vape_naysh (Autodesk Fusion 360 design; units mm, degrees)
Autodesk Fusion 360 part; units mm, degrees
(part 1 of 3)
sketch "Sketch1" plane through (0, 0, 0) normal (0, 1, 0) x (1, 0, 0)
  line L0 (3, -30) -> (14, -30)
  line L1 (14, -30) -> (16, -17)
  line L2 (16, -17) -> (19.2504, -13.3707)
  line L3 (19.2504, -13.3707) -> (19.2504, 30)
  line L4 (19.2504, 30) -> (15, 34.5)
  line L5 (15, 34.5) -> (-12.65, 34.5)
  line L6 (-12.65, 34.5) -> (-16.7887, 30.816)
  line L7 (-16.7887, 30.816) -> (-16.7887, -12.5)
  line L8 (-16.7887, -12.5) -> (-14, -16.5)
  line L9 (-14, -16.5) -> (-1, -16.5)
  line L10 (-1, -16.5) -> (1.175, -18.2567)
  line L11 (1.175, -18.2567) -> (3, -30)
  line L12 (14.6863, -30.8) -> (16.7545, -17.3566)
  line L13 (16.7545, -17.3566) -> (20.0504, -13.6766)
  line L14 (20.0504, -13.6766) -> (20.0504, 30.3181)
  line L15 (20.0504, 30.3181) -> (15.3448, 35.3)
  line L16 (15.3448, 35.3) -> (-12.9545, 35.3)
  line L17 (-12.9545, 35.3) -> (-17.5887, 31.1749)
  line L18 (-17.5887, 31.1749) -> (-17.5887, -12.7513)
  line L19 (-17.5887, -12.7513) -> (-14.4175, -17.3)
  line L20 (-14.4175, -17.3) -> (-1.2827, -17.3)
  line L21 (-1.2827, -17.3) -> (0.4319, -18.6849)
  line L22 (0.4319, -18.6849) -> (2.3147, -30.8)
  line L23 (2.3147, -30.8) -> (14.6863, -30.8)
  dimension "d1" = 0.8
  constraint horizontal L0
  constraint perpendicular L0 L3
  constraint perpendicular L3 L5
  constraint perpendicular L5 L7
  constraint perpendicular L3 L9
sketch "Sketch2" plane through (0, 0, 0) normal (0, 1, 0) x (1, 0, 0)
  spline S0 degree 3 poles (-4.3083, 22.4434) (-8.6322, 22.1667) (-11.0016, 21.717) (-11.5724, 21.0771) knots 0 0 0 0 1 1 1 1
  spline S1 degree 3 poles (-11.5724, 21.0771) (-11.7799, 20.8349) (-11.8491, 20.5236) (-11.8145, 19.9183) knots 0 0 0 0 1 1 1 1
  spline S2 degree 3 poles (-11.8145, 19.9183) (-11.7626, 19.1054) (-11.728, 19.0535) (-10.9843, 18.6903) knots 0 0 0 0 1 1 1 1
  spline S3 degree 3 poles (-10.9843, 18.6903) (-10.2579, 18.3271) (-9.3067, 18.1714) (-4.6715, 17.6526) knots 0 0 0 0 1 1 1 1
  line L0 (-4.6715, 17.6526) -> (-3.4608, 17.5142)
  line L1 (-3.4608, 17.5142) -> (-2.9074, 16.1306)
  spline S4 degree 3 poles (-2.9074, 16.1306) (-2.6133, 15.3696) (-2.3193, 14.4875) (-2.2501, 14.1935) knots 0 0 0 0 1 1 1 1
  line L2 (-2.2501, 14.1935) -> (-2.1291, 13.6228)
  line L3 (-2.1291, 13.6228) -> (-3.236, 13.6228)
  spline S5 degree 3 poles (-3.236, 13.6228) (-4.5331, 13.6228) (-7.7674, 13.2077) (-8.4073, 12.9655) knots 0 0 0 0 1 1 1 1
  spline S6 degree 3 poles (-8.4073, 12.9655) (-9.1337, 12.6715) (-9.4277, 12.2737) (-9.4277, 11.53) knots 0 0 0 0 1 1 1 1
  spline S7 degree 3 poles (-9.4277, 11.53) (-9.4277, 10.1291) (-8.3381, 9.7659) (-2.9766, 9.3681) knots 0 0 0 0 1 1 1 1
  spline S8 degree 3 poles (-2.9766, 9.3681) (-2.1464, 9.3162) (-1.4719, 9.1951) (-1.4719, 9.1259) knots 0 0 0 0 1 1 1 1
  spline S9 degree 3 poles (-1.4719, 9.1259) (-1.4719, 9.0395) (-1.8351, 9.0049) (-2.2847, 9.0741) knots 0 0 0 0 1 1 1 1
  spline S10 degree 3 poles (-2.2847, 9.0741) (-3.4435, 9.1951) (-4.5504, 8.8665) (-5.2077, 8.1747) knots 0 0 0 0 1 1 1 1
  spline S11 degree 3 poles (-5.2077, 8.1747) (-5.7092, 7.6385) (-5.813, 7.6039) (-7.1102, 7.5521) knots 0 0 0 0 1 1 1 1
  spline S12 degree 3 poles (-7.1102, 7.5521) (-8.2862, 7.5002) (-8.6149, 7.4137) (-9.2375, 6.9986) knots 0 0 0 0 1 1 1 1
  spline S13 degree 3 poles (-9.2375, 6.9986) (-10.0158, 6.4797) (-10.6211, 5.4247) (-10.6384, 4.6118) knots 0 0 0 0 1 1 1 1
  spline S14 degree 3 poles (-10.6384, 4.6118) (-10.6384, 4.3524) (-10.7595, 4.0584) (-10.9152, 3.92) knots 0 0 0 0 1 1 1 1
  spline S15 degree 3 poles (-10.9152, 3.92) (-11.5724, 3.3666) (-11.9183, 2.3288) (-11.9356, 0.8241) knots 0 0 0 0 1 1 1 1
  spline S16 degree 3 poles (-11.9356, 0.8241) (-11.9356, -0.94) (-11.607, -1.7529) (-10.6211, -2.4447) knots 0 0 0 0 1 1 1 1
  spline S17 degree 3 poles (-10.6211, -2.4447) (-10.2579, -2.6868) (-9.9639, -3.0154) (-9.9466, -3.1538) knots 0 0 0 0 1 1 1 1
  spline S18 degree 3 poles (-9.9466, -3.1538) (-9.9466, -3.2922) (-9.7909, -3.6727) (-9.6007, -3.984) knots 0 0 0 0 1 1 1 1
  spline S19 degree 3 poles (-9.6007, -3.984) (-9.4104, -4.2953) (-9.2548, -4.7277) (-9.2548, -4.9352) knots 0 0 0 0 1 1 1 1
  spline S20 degree 3 poles (-9.2548, -4.9352) (-9.2548, -5.506) (-8.4938, -6.5264) (-7.8193, -6.855) knots 0 0 0 0 1 1 1 1
  spline S21 degree 3 poles (-7.8193, -6.855) (-7.4907, -7.0107) (-6.8334, -7.1317) (-6.3665, -7.1317) knots 0 0 0 0 1 1 1 1
  spline S22 degree 3 poles (-6.3665, -7.1317) (-5.9168, -7.1317) (-5.225, -7.2528) (-4.8445, -7.3912) knots 0 0 0 0 1 1 1 1
  spline S23 degree 3 poles (-4.8445, -7.3912) (-4.464, -7.5295) (-3.9105, -7.6333) (-3.6165, -7.6506) knots 0 0 0 0 1 1 1 1
  spline S24 degree 3 poles (-3.6165, -7.6506) (-3.3052, -7.6506) (-3.0284, -7.7544) (-2.9766, -7.8927) knots 0 0 0 0 1 1 1 1
  spline S25 degree 3 poles (-2.9766, -7.8927) (-2.9247, -8.0311) (-2.5096, -8.3597) (-2.0426, -8.6364) knots 0 0 0 0 1 1 1 1
  spline S26 degree 3 poles (-2.0426, -8.6364) (-1.2989, -9.0688) (-1.0395, -9.1207) (0.2577, -9.1207) knots 0 0 0 0 1 1 1 1
  spline S27 degree 3 poles (0.2577, -9.1207) (1.9008, -9.1207) (2.4888, -8.8959) (3.4919, -7.8927) knots 0 0 0 0 1 1 1 1
  spline S28 degree 3 poles (3.4919, -7.8927) (3.8033, -7.5641) (4.2356, -7.3047) (4.4259, -7.3047) knots 0 0 0 0 1 1 1 1
  spline S29 degree 3 poles (4.4259, -7.3047) (4.6334, -7.3047) (5.2388, -7.0799) (5.7749, -6.8031) knots 0 0 0 0 1 1 1 1
  spline S30 degree 3 poles (5.7749, -6.8031) (6.5013, -6.4226) (7.0721, -6.267) (8.0406, -6.1978) knots 0 0 0 0 1 1 1 1
  spline S31 degree 3 poles (8.0406, -6.1978) (10.4966, -6.0075) (11.7591, -5.8173) (12.1223, -5.5925) knots 0 0 0 0 1 1 1 1
  spline S32 degree 3 poles (12.1223, -5.5925) (12.745, -5.1947) (13.0909, -4.3991) (13.2465, -3.05) knots 0 0 0 0 1 1 1 1
  spline S33 degree 3 poles (13.2465, -3.05) (13.3676, -2.0988) (13.5579, -1.5626) (13.973, -0.8881) knots 0 0 0 0 1 1 1 1
  spline S34 degree 3 poles (13.973, -0.8881) (14.4918, -0.0579) (14.5264, 0.1323) (14.5264, 1.516) knots 0 0 0 0 1 1 1 1
  spline S35 degree 3 poles (14.5264, 1.516) (14.5264, 2.865) (14.4745, 3.0898) (14.0594, 3.7298) knots 0 0 0 0 1 1 1 1
  spline S36 degree 3 poles (14.0594, 3.7298) (13.8, 4.1276) (13.2638, 4.6291) (12.8833, 4.8367) knots 0 0 0 0 1 1 1 1
  spline S37 degree 3 poles (12.8833, 4.8367) (12.451, 5.0961) (12.1915, 5.3555) (12.1915, 5.5804) knots 0 0 0 0 1 1 1 1
  spline S38 degree 3 poles (12.1915, 5.5804) (12.1915, 6.1165) (11.5689, 7.0159) (10.9463, 7.4137) knots 0 0 0 0 1 1 1 1
  spline S39 degree 3 poles (10.9463, 7.4137) (10.4447, 7.7077) (10.1853, 7.7423) (8.8189, 7.6731) knots 0 0 0 0 1 1 1 1
  spline S40 degree 3 poles (8.8189, 7.6731) (6.5359, 7.5348) (5.5501, 7.5694) (5.4117, 7.7942) knots 0 0 0 0 1 1 1 1
  spline S41 degree 3 poles (5.4117, 7.7942) (5.3425, 7.9153) (5.2734, 8.2785) (5.2734, 8.6417) knots 0 0 0 0 1 1 1 1
  line L4 (5.2734, 8.6417) -> (5.2734, 9.2643)
  line L5 (5.2734, 9.2643) -> (6.6224, 9.3681)
  spline S42 degree 3 poles (6.6224, 9.3681) (11.3613, 9.7486) (12.5374, 10.1637) (12.5374, 11.4781) knots 0 0 0 0 1 1 1 1
  spline S43 degree 3 poles (12.5374, 11.4781) (12.5374, 12.3083) (12.2953, 12.6888) (11.6381, 12.9136) knots 0 0 0 0 1 1 1 1
  spline S44 degree 3 poles (11.6381, 12.9136) (10.8771, 13.1904) (7.8331, 13.6228) (6.6916, 13.6228) knots 0 0 0 0 1 1 1 1
  spline S45 degree 3 poles (6.6916, 13.6228) (5.896, 13.6228) (5.7749, 13.6573) (5.8441, 13.9341) knots 0 0 0 0 1 1 1 1
  spline S46 degree 3 poles (5.8441, 13.9341) (6.2938, 15.5425) (6.7089, 16.7359) (7.0029, 17.2202) knots 0 0 0 0 1 1 1 1
  spline S47 degree 3 poles (7.0029, 17.2202) (7.3142, 17.7218) (7.418, 17.7737) (8.1617, 17.7737) knots 0 0 0 0 1 1 1 1
  spline S48 degree 3 poles (8.1617, 17.7737) (9.1994, 17.7737) (12.3472, 18.2233) (13.2465, 18.4828) knots 0 0 0 0 1 1 1 1
  spline S49 degree 3 poles (13.2465, 18.4828) (14.2324, 18.7941) (14.4745, 19.1227) (14.4053, 20.2123) knots 0 0 0 0 1 1 1 1
  spline S50 degree 3 poles (14.4053, 20.2123) (14.3535, 21.0252) (14.3016, 21.1636) (13.8865, 21.3711) knots 0 0 0 0 1 1 1 1
  spline S51 degree 3 poles (13.8865, 21.3711) (13.2465, 21.6651) (11.4478, 22.0283) (9.4243, 22.2705) knots 0 0 0 0 1 1 1 1
  spline S52 degree 3 poles (9.4243, 22.2705) (7.245, 22.5126) (-1.5064, 22.6337) (-4.3083, 22.4434) knots 0 0 0 0 1 1 1 1
  spline S53 degree 3 poles (5.2734, 20.368) (6.2765, 20.3161) (6.8818, 20.2469) (6.6397, 20.2296) knots 0 0 0 0 1 1 1 1
  spline S54 degree 3 poles (6.6397, 20.2296) (5.8787, 20.1777) (5.1004, 19.1227) (4.3913, 17.1856) knots 0 0 0 0 1 1 1 1
  line L6 (4.3913, 17.1856) -> (4.0627, 16.3035)
  line L7 (4.0627, 16.3035) -> (4.1665, 17.1164)
  spline S55 degree 3 poles (4.1665, 17.1164) (4.2356, 17.5661) (4.2183, 18.1369) (4.1665, 18.379) knots 0 0 0 0 1 1 1 1
  spline S56 degree 3 poles (4.1665, 18.379) (4.0627, 18.7768) (3.9762, 18.8114) (3.1979, 18.8114) knots 0 0 0 0 1 1 1 1
  spline S57 degree 3 poles (3.1979, 18.8114) (2.4196, 18.8114) (2.2985, 18.7595) (2.1602, 18.3617) knots 0 0 0 0 1 1 1 1
  spline S58 degree 3 poles (2.1602, 18.3617) (2.0564, 18.1196) (1.9872, 17.7045) (1.9872, 17.4277) knots 0 0 0 0 1 1 1 1
  spline S59 degree 3 poles (1.9872, 17.4277) (1.9872, 17.151) (1.918, 16.8916) (1.8316, 16.8397) knots 0 0 0 0 1 1 1 1
  spline S60 degree 3 poles (1.8316, 16.8397) (1.7624, 16.7878) (1.6413, 17.4104) (1.5721, 18.2406) knots 0 0 0 0 1 1 1 1
  spline S61 degree 3 poles (1.5721, 18.2406) (1.3992, 20.2469) (1.3127, 20.4026) (0.2923, 20.3334) knots 0 0 0 0 1 1 1 1
  line L8 (0.2923, 20.3334) -> (-0.5206, 20.2815)
  line L9 (-0.5206, 20.2815) -> (-0.486, 18.4136)
  line L10 (-0.486, 18.4136) -> (-0.4687, 16.5284)
  line L11 (-0.4687, 16.5284) -> (-1.0395, 17.8428)
  spline S62 degree 3 poles (-1.0395, 17.8428) (-1.3508, 18.5519) (-1.7659, 19.4167) (-1.9561, 19.7453) knots 0 0 0 0 1 1 1 1
  line L12 (-1.9561, 19.7453) -> (-2.3193, 20.3507)
  line L13 (-2.3193, 20.3507) -> (-1.7659, 20.4198)
  spline S63 degree 3 poles (-1.7659, 20.4198) (-0.8492, 20.5236) (3.3363, 20.5063) (5.2734, 20.368) knots 0 0 0 0 1 1 1 1
  spline S64 degree 3 poles (-4.1008, 20.1604) (-4.2045, 19.8491) (-4.6542, 19.7972) (-5.6055, 19.9529) knots 0 0 0 0 1 1 1 1
  line L14 (-5.6055, 19.9529) -> (-6.401, 20.0912)
  line L15 (-6.401, 20.0912) -> (-5.3633, 20.2123)
  spline S65 degree 3 poles (-5.3633, 20.2123) (-4.7926, 20.2642) (-4.2564, 20.3161) (-4.1872, 20.3334) knots 0 0 0 0 1 1 1 1
  spline S66 degree 3 poles (-4.1872, 20.3334) (-4.1008, 20.3507) (-4.0662, 20.2642) (-4.1008, 20.1604) knots 0 0 0 0 1 1 1 1
  spline S67 degree 3 poles (8.8189, 20.0221) (8.767, 19.9356) (8.4903, 19.8491) (8.2136, 19.8491) knots 0 0 0 0 1 1 1 1
  spline S68 degree 3 poles (8.2136, 19.8491) (7.9369, 19.8491) (7.6601, 19.9356) (7.6082, 20.0221) knots 0 0 0 0 1 1 1 1
  spline S69 degree 3 poles (7.6082, 20.0221) (7.5391, 20.1258) (7.7812, 20.195) (8.2136, 20.195) knots 0 0 0 0 1 1 1 1
  spline S70 degree 3 poles (8.2136, 20.195) (8.646, 20.195) (8.8881, 20.1258) (8.8189, 20.0221) knots 0 0 0 0 1 1 1 1
  spline S71 degree 3 poles (1.4684, 9.2297) (1.4684, 8.6936) (1.3819, 8.4341) (1.1916, 8.3649) knots 0 0 0 0 1 1 1 1
  spline S72 degree 3 poles (1.1916, 8.3649) (0.6728, 8.1747) (0.6036, 8.2612) (0.6036, 9.1259) knots 0 0 0 0 1 1 1 1
  spline S73 degree 3 poles (0.6036, 9.1259) (0.6036, 9.9388) (0.6382, 9.9907) (1.036, 9.9907) knots 0 0 0 0 1 1 1 1
  spline S74 degree 3 poles (1.036, 9.9907) (1.4338, 9.9907) (1.4684, 9.9215) (1.4684, 9.2297) knots 0 0 0 0 1 1 1 1
  spline S75 degree 3 poles (-0.2266, 5.148) (-0.2612, 4.7502) (-0.2093, 4.3351) (-0.0882, 4.1967) knots 0 0 0 0 1 1 1 1
  spline S76 degree 3 poles (-0.0882, 4.1967) (0.2404, 3.8163) (1.3473, 3.8681) (1.8835, 4.3005) knots 0 0 0 0 1 1 1 1
  spline S77 degree 3 poles (1.8835, 4.3005) (2.3504, 4.6637) (2.3677, 4.6637) (2.8001, 4.3524) knots 0 0 0 0 1 1 1 1
  spline S78 degree 3 poles (2.8001, 4.3524) (3.0423, 4.1622) (3.3363, 3.7471) (3.44, 3.4185) knots 0 0 0 0 1 1 1 1
  spline S79 degree 3 poles (3.44, 3.4185) (3.6303, 2.8304) (3.6649, 2.8131) (4.4951, 2.8131) knots 0 0 0 0 1 1 1 1
  line L16 (4.4951, 2.8131) -> (5.3598, 2.8131)
  line L17 (5.3598, 2.8131) -> (5.4117, 3.799)
  spline S80 degree 3 poles (5.4117, 3.799) (5.4463, 4.3524) (5.3771, 4.9577) (5.2734, 5.148) knots 0 0 0 0 1 1 1 1
  spline S81 degree 3 poles (5.2734, 5.148) (5.135, 5.4247) (5.135, 5.4939) (5.3425, 5.4939) knots 0 0 0 0 1 1 1 1
  spline S82 degree 3 poles (5.3425, 5.4939) (6.2073, 5.4939) (7.8504, 4.2486) (7.5045, 3.8335) knots 0 0 0 0 1 1 1 1
  spline S83 degree 3 poles (7.5045, 3.8335) (7.418, 3.7125) (7.3488, 3.2455) (7.3834, 2.7785) knots 0 0 0 0 1 1 1 1
  line L18 (7.3834, 2.7785) -> (7.4353, 1.9483)
  line L19 (7.4353, 1.9483) -> (8.2309, 1.8965)
  spline S84 degree 3 poles (8.2309, 1.8965) (8.94, 1.8446) (9.0956, 1.9138) (9.6491, 2.4672) knots 0 0 0 0 1 1 1 1
  spline S85 degree 3 poles (9.6491, 2.4672) (10.4793, 3.2974) (11.1019, 3.2974) (11.8629, 2.4326) knots 0 0 0 0 1 1 1 1
  line L20 (11.8629, 2.4326) -> (12.4337, 1.7754)
  line L21 (12.4337, 1.7754) -> (11.4478, 1.7235)
  line L22 (11.4478, 1.7235) -> (10.462, 1.6716)
  line L23 (10.462, 1.6716) -> (10.462, 0.8241)
  spline S86 degree 3 poles (10.462, 0.8241) (10.462, 0.1496) (10.5485, -0.1098) (10.8944, -0.4557) knots 0 0 0 0 1 1 1 1
  spline S87 degree 3 poles (10.8944, -0.4557) (11.4305, -0.9919) (11.4305, -1.2686) (10.9463, -1.7356) knots 0 0 0 0 1 1 1 1
  spline S88 degree 3 poles (10.9463, -1.7356) (10.6522, -1.995) (10.2717, -2.1161) (9.5972, -2.1507) knots 0 0 0 0 1 1 1 1
  line L24 (9.5972, -2.1507) -> (8.646, -2.2026)
  line L25 (8.646, -2.2026) -> (8.5595, -3.1538)
  spline S89 degree 3 poles (8.5595, -3.1538) (8.473, -4.0359) (8.4384, -4.1051) (7.9023, -4.2607) knots 0 0 0 0 1 1 1 1
  spline S90 degree 3 poles (7.9023, -4.2607) (7.1759, -4.4683) (7.0894, -4.3472) (7.4353, -3.6727) knots 0 0 0 0 1 1 1 1
  spline S91 degree 3 poles (7.4353, -3.6727) (7.6082, -3.3268) (7.6947, -2.8252) (7.6601, -2.2371) knots 0 0 0 0 1 1 1 1
  line L26 (7.6601, -2.2371) -> (7.6082, -1.3378)
  line L27 (7.6082, -1.3378) -> (6.7262, -1.2859)
  spline S92 degree 3 poles (6.7262, -1.2859) (5.896, -1.234) (5.8441, -1.2513) (5.602, -1.7875) knots 0 0 0 0 1 1 1 1
  spline S93 degree 3 poles (5.602, -1.7875) (5.4809, -2.0988) (5.1523, -2.4966) (4.8929, -2.6868) knots 0 0 0 0 1 1 1 1
  spline S94 degree 3 poles (4.8929, -2.6868) (4.4605, -3.0154) (4.4086, -3.0154) (3.9935, -2.756) knots 0 0 0 0 1 1 1 1
  spline S95 degree 3 poles (3.9935, -2.756) (3.7514, -2.5831) (3.2152, -2.462) (2.7828, -2.462) knots 0 0 0 0 1 1 1 1
  spline S96 degree 3 poles (2.7828, -2.462) (1.9526, -2.462) (1.8143, -2.6176) (1.8143, -3.5689) knots 0 0 0 0 1 1 1 1
  spline S97 degree 3 poles (1.8143, -3.5689) (1.8143, -4.2607) (2.2121, -4.6585) (3.2325, -4.9698) knots 0 0 0 0 1 1 1 1
  line L28 (3.2325, -4.9698) -> (3.9762, -5.1774)
  line L29 (3.9762, -5.1774) -> (3.3363, -5.3676)
  spline S98 degree 3 poles (3.3363, -5.3676) (2.9904, -5.4541) (2.4542, -5.4887) (2.1429, -5.4195) knots 0 0 0 0 1 1 1 1
  line L30 (2.1429, -5.4195) -> (1.5721, -5.2984)
  line L31 (1.5721, -5.2984) -> (1.624, -4.2434)
  spline S99 degree 3 poles (1.624, -4.2434) (1.6586, -3.223) (1.6413, -3.1538) (1.2435, -3.0673) knots 0 0 0 0 1 1 1 1
  spline S100 degree 3 poles (1.2435, -3.0673) (0.4134, -2.8598) (-0.1574, -3.0327) (-0.4168, -3.5862) knots 0 0 0 0 1 1 1 1
  spline S101 degree 3 poles (-0.4168, -3.5862) (-1.0741, -5.0217) (-2.475, -5.8173) (-3.5473, -5.3503) knots 0 0 0 0 1 1 1 1
  line L32 (-3.5473, -5.3503) -> (-4.1526, -5.0909)
  line L33 (-4.1526, -5.0909) -> (-3.5127, -5.0736)
  spline S102 degree 3 poles (-3.5127, -5.0736) (-3.1668, -5.0563) (-2.6652, -4.9698) (-2.4231, -4.8488) knots 0 0 0 0 1 1 1 1
  spline S103 degree 3 poles (-2.4231, -4.8488) (-2.008, -4.6585) (-1.9734, -4.572) (-2.0253, -3.7764) knots 0 0 0 0 1 1 1 1
  line L34 (-2.0253, -3.7764) -> (-2.0772, -2.8944)
  line L35 (-2.0772, -2.8944) -> (-3.1668, -2.8771)
  spline S104 degree 3 poles (-3.1668, -2.8771) (-4.4294, -2.8425) (-4.8963, -2.5312) (-5.0866, -1.5799) knots 0 0 0 0 1 1 1 1
  spline S105 degree 3 poles (-5.0866, -1.5799) (-5.1904, -1.0265) (-5.2422, -0.9919) (-6.0378, -0.94) knots 0 0 0 0 1 1 1 1
  spline S106 degree 3 poles (-6.0378, -0.94) (-6.4875, -0.9054) (-6.9718, -0.9746) (-7.0929, -1.0784) knots 0 0 0 0 1 1 1 1
  spline S107 degree 3 poles (-7.0929, -1.0784) (-7.4734, -1.3897) (-8.3554, -1.1129) (-8.9954, -0.4557) knots 0 0 0 0 1 1 1 1
  spline S108 degree 3 poles (-8.9954, -0.4557) (-9.7909, 0.3226) (-9.912, 0.8933) (-9.4969, 1.6716) knots 0 0 0 0 1 1 1 1
  spline S109 degree 3 poles (-9.4969, 1.6716) (-8.9608, 2.6402) (-8.4246, 2.9342) (-7.0756, 2.9688) knots 0 0 0 0 1 1 1 1
  line L36 (-7.0756, 2.9688) -> (-5.8822, 2.9861)
  line L37 (-5.8822, 2.9861) -> (-5.8303, 3.7817)
  spline S110 degree 3 poles (-5.8303, 3.7817) (-5.7784, 4.4908) (-5.7092, 4.6291) (-5.2768, 4.8021) knots 0 0 0 0 1 1 1 1
  spline S111 degree 3 poles (-5.2768, 4.8021) (-4.8963, 4.9577) (-4.7061, 4.9577) (-4.3429, 4.7675) knots 0 0 0 0 1 1 1 1
  line L38 (-4.3429, 4.7675) -> (-3.8932, 4.5254)
  line L39 (-3.8932, 4.5254) -> (-4.4985, 4.214)
  spline S112 degree 3 poles (-4.4985, 4.214) (-5.1904, 3.8335) (-5.7957, 2.7439) (-5.7957, 1.8446) knots 0 0 0 0 1 1 1 1
  spline S113 degree 3 poles (-5.7957, 1.8446) (-5.7957, 1.0836) (-5.5363, 0.8241) (-4.758, 0.8241) knots 0 0 0 0 1 1 1 1
  spline S114 degree 3 poles (-4.758, 0.8241) (-4.0316, 0.8241) (-3.8932, 0.9279) (-3.5473, 1.5851) knots 0 0 0 0 1 1 1 1
  spline S115 degree 3 poles (-3.5473, 1.5851) (-3.4089, 1.8619) (-3.1149, 2.1905) (-2.9247, 2.3288) knots 0 0 0 0 1 1 1 1
  spline S116 degree 3 poles (-2.9247, 2.3288) (-2.596, 2.5364) (-2.4923, 2.5191) (-2.0253, 2.1213) knots 0 0 0 0 1 1 1 1
  spline S117 degree 3 poles (-2.0253, 2.1213) (-1.4546, 1.6543) (-0.3304, 1.516) (0.0501, 1.8965) knots 0 0 0 0 1 1 1 1
  spline S118 degree 3 poles (0.0501, 1.8965) (0.6382, 2.4845) (0.0156, 3.9373) (-1.0049, 4.3697) knots 0 0 0 0 1 1 1 1
  line L40 (-1.0049, 4.3697) -> (-1.5064, 4.5772)
  line L41 (-1.5064, 4.5772) -> (-0.953, 5.2172)
  spline S119 degree 3 poles (-0.953, 5.2172) (-0.6417, 5.5631) (-0.3476, 5.8398) (-0.2785, 5.8398) knots 0 0 0 0 1 1 1 1
  spline S120 degree 3 poles (-0.2785, 5.8398) (-0.2093, 5.8398) (-0.192, 5.5285) (-0.2266, 5.148) knots 0 0 0 0 1 1 1 1
  line L42 (-16, 6.7046) -> (-16, -10.5908)
  line L43 (-16, -10.5908) -> (1.2954, -10.5908)
  line L44 (1.2954, -10.5908) -> (18.5908, -10.5908)
  line L45 (18.5908, -10.5908) -> (18.5908, 6.7046)
  line L46 (18.5908, 6.7046) -> (18.5908, 24)
  line L47 (18.5908, 24) -> (1.2954, 24)
  line L48 (1.2954, 24) -> (-16, 24)
  line L49 (-16, 24) -> (-16, 6.7046)
  spline S121 degree 3 poles (8.9054, 21.7343) (10.9117, 21.5095) (12.7277, 21.1463) (13.3676, 20.8522) knots 0 0 0 0 1 1 1 1
  spline S122 degree 3 poles (13.3676, 20.8522) (13.9384, 20.5755) (14.0767, 19.8664) (13.627, 19.4513) knots 0 0 0 0 1 1 1 1
  spline S123 degree 3 poles (13.627, 19.4513) (13.0736, 18.967) (10.7906, 18.5346) (7.2623, 18.2406) knots 0 0 0 0 1 1 1 1
  spline S124 degree 3 poles (7.2623, 18.2406) (6.8645, 18.2233) (6.6743, 18.0504) (6.363, 17.5142) knots 0 0 0 0 1 1 1 1
  spline S125 degree 3 poles (6.363, 17.5142) (5.9825, 16.8224) (5.3425, 14.6605) (5.2388, 13.7092) knots 0 0 0 0 1 1 1 1
  spline S126 degree 3 poles (5.2388, 13.7092) (5.1869, 13.2077) (5.2215, 13.1904) (5.8787, 13.1558) knots 0 0 0 0 1 1 1 1
  spline S127 degree 3 poles (5.8787, 13.1558) (7.4872, 13.052) (9.9258, 12.7234) (10.756, 12.4813) knots 0 0 0 0 1 1 1 1
  spline S128 degree 3 poles (10.756, 12.4813) (12.1223, 12.1008) (12.3645, 11.3052) (11.3095, 10.7517) knots 0 0 0 0 1 1 1 1
  spline S129 degree 3 poles (11.3095, 10.7517) (10.756, 10.475) (8.2136, 10.0599) (6.1035, 9.8869) knots 0 0 0 0 1 1 1 1
  line L50 (6.1035, 9.8869) -> (4.7891, 9.7832)
  line L51 (4.7891, 9.7832) -> (4.7199, 8.7281)
  spline S130 degree 3 poles (4.7199, 8.7281) (4.6507, 7.431) (4.8237, 7.0505) (5.5501, 7.0505) knots 0 0 0 0 1 1 1 1
  spline S131 degree 3 poles (5.5501, 7.0505) (5.8441, 7.0505) (6.3284, 6.964) (6.6397, 6.8602) knots 0 0 0 0 1 1 1 1
  spline S132 degree 3 poles (6.6397, 6.8602) (7.0721, 6.7046) (7.2969, 6.7219) (7.7639, 6.9467) knots 0 0 0 0 1 1 1 1
  spline S133 degree 3 poles (7.7639, 6.9467) (8.5768, 7.3272) (9.7356, 7.2926) (10.4274, 6.8775) knots 0 0 0 0 1 1 1 1
  spline S134 degree 3 poles (10.4274, 6.8775) (11.05, 6.497) (11.6727, 5.5977) (11.6727, 5.0615) knots 0 0 0 0 1 1 1 1
  spline S135 degree 3 poles (11.6727, 5.0615) (11.6727, 4.8367) (11.9321, 4.5772) (12.3645, 4.3178) knots 0 0 0 0 1 1 1 1
  spline S136 degree 3 poles (12.3645, 4.3178) (14.0248, 3.3839) (14.4918, 1.3949) (13.4887, -0.3001) knots 0 0 0 0 1 1 1 1
  spline S137 degree 3 poles (13.4887, -0.3001) (12.8833, -1.3032) (12.6758, -1.9777) (12.6931, -2.7906) knots 0 0 0 0 1 1 1 1
  spline S138 degree 3 poles (12.6931, -2.7906) (12.7277, -3.6035) (12.1396, -4.745) (11.4997, -5.1082) knots 0 0 0 0 1 1 1 1
  spline S139 degree 3 poles (11.4997, -5.1082) (11.1538, -5.3157) (10.6868, -5.4195) (10.1507, -5.3849) knots 0 0 0 0 1 1 1 1
  spline S140 degree 3 poles (10.1507, -5.3849) (9.701, -5.3676) (9.1129, -5.4541) (8.8189, -5.5579) knots 0 0 0 0 1 1 1 1
  spline S141 degree 3 poles (8.8189, -5.5579) (8.5422, -5.6789) (7.8158, -5.7481) (7.245, -5.7135) knots 0 0 0 0 1 1 1 1
  spline S142 degree 3 poles (7.245, -5.7135) (6.6397, -5.6962) (6.0862, -5.7481) (5.9479, -5.8519) knots 0 0 0 0 1 1 1 1
  spline S143 degree 3 poles (5.9479, -5.8519) (5.4982, -6.2151) (4.2529, -6.7858) (3.907, -6.7858) knots 0 0 0 0 1 1 1 1
  spline S144 degree 3 poles (3.907, -6.7858) (3.7168, -6.7858) (3.2844, -7.0453) (2.9731, -7.3739) knots 0 0 0 0 1 1 1 1
  spline S145 degree 3 poles (2.9731, -7.3739) (1.624, -8.7229) (-0.0363, -8.9824) (-1.5237, -8.1176) knots 0 0 0 0 1 1 1 1
  spline S146 degree 3 poles (-1.5237, -8.1176) (-1.9907, -7.8409) (-2.4058, -7.5122) (-2.4577, -7.3739) knots 0 0 0 0 1 1 1 1
  spline S147 degree 3 poles (-2.4577, -7.3739) (-2.5096, -7.2355) (-2.7863, -7.1317) (-3.0976, -7.1317) knots 0 0 0 0 1 1 1 1
  spline S148 degree 3 poles (-3.0976, -7.1317) (-3.3916, -7.1145) (-3.9451, -6.9934) (-4.3256, -6.8377) knots 0 0 0 0 1 1 1 1
  spline S149 degree 3 poles (-4.3256, -6.8377) (-4.7061, -6.6994) (-5.3806, -6.5956) (-5.8303, -6.5956) knots 0 0 0 0 1 1 1 1
  spline S150 degree 3 poles (-5.8303, -6.5956) (-6.2973, -6.6129) (-6.9199, -6.5091) (-7.2831, -6.3362) knots 0 0 0 0 1 1 1 1
  spline S151 degree 3 poles (-7.2831, -6.3362) (-7.9749, -6.0075) (-8.7359, -5.0044) (-8.7359, -4.4164) knots 0 0 0 0 1 1 1 1
  spline S152 degree 3 poles (-8.7359, -4.4164) (-8.7359, -4.2088) (-8.8916, -3.7764) (-9.0818, -3.4651) knots 0 0 0 0 1 1 1 1
  spline S153 degree 3 poles (-9.0818, -3.4651) (-9.2721, -3.1538) (-9.4277, -2.7733) (-9.4277, -2.6349) knots 0 0 0 0 1 1 1 1
  spline S154 degree 3 poles (-9.4277, -2.6349) (-9.445, -2.4966) (-9.7391, -2.168) (-10.1023, -1.9258) knots 0 0 0 0 1 1 1 1
  spline S155 degree 3 poles (-10.1023, -1.9258) (-10.9497, -1.3205) (-11.3994, -0.3865) (-11.3994, 0.8241) knots 0 0 0 0 1 1 1 1
  spline S156 degree 3 poles (-11.3994, 0.8241) (-11.3821, 1.7927) (-10.9324, 2.9515) (-10.3963, 3.4012) knots 0 0 0 0 1 1 1 1
  spline S157 degree 3 poles (-10.3963, 3.4012) (-10.2406, 3.5395) (-10.1196, 3.8335) (-10.1196, 4.093) knots 0 0 0 0 1 1 1 1
  spline S158 degree 3 poles (-10.1196, 4.093) (-10.1023, 4.9059) (-9.4969, 5.9609) (-8.7186, 6.4797) knots 0 0 0 0 1 1 1 1
  spline S159 degree 3 poles (-8.7186, 6.4797) (-8.1306, 6.8775) (-7.802, 6.964) (-7.0237, 6.9467) knots 0 0 0 0 1 1 1 1
  spline S160 degree 3 poles (-7.0237, 6.9467) (-6.4875, 6.9467) (-5.8995, 6.8948) (-5.7092, 6.8257) knots 0 0 0 0 1 1 1 1
  spline S161 degree 3 poles (-5.7092, 6.8257) (-5.4325, 6.7219) (-5.2768, 6.8257) (-4.9828, 7.2926) knots 0 0 0 0 1 1 1 1
  spline S162 degree 3 poles (-4.9828, 7.2926) (-4.2564, 8.4168) (-2.7171, 8.8146) (-1.5064, 8.192) knots 0 0 0 0 1 1 1 1
  line L52 (-1.5064, 8.192) -> (-0.953, 7.898)
  line L53 (-0.953, 7.898) -> (-0.953, 8.8492)
  line L54 (-0.953, 8.8492) -> (-0.953, 9.7832)
  line L55 (-0.953, 9.7832) -> (-2.4577, 9.8869)
  spline S163 degree 3 poles (-2.4577, 9.8869) (-4.9309, 10.0599) (-7.6463, 10.475) (-8.1825, 10.7517) knots 0 0 0 0 1 1 1 1
  spline S164 degree 3 poles (-8.1825, 10.7517) (-9.0991, 11.236) (-9.0818, 11.8586) (-8.1133, 12.3256) knots 0 0 0 0 1 1 1 1
  spline S165 degree 3 poles (-8.1133, 12.3256) (-7.4388, 12.6369) (-4.3083, 13.1039) (-2.7171, 13.1039) knots 0 0 0 0 1 1 1 1
  spline S166 degree 3 poles (-2.7171, 13.1039) (-1.8869, 13.1039) (-1.6102, 13.1731) (-1.5237, 13.3806) knots 0 0 0 0 1 1 1 1
  spline S167 degree 3 poles (-1.5237, 13.3806) (-1.4027, 13.6919) (-2.008, 15.8539) (-2.5961, 17.1683) knots 0 0 0 0 1 1 1 1
  line L56 (-2.5961, 17.1683) -> (-2.9939, 18.085)
  line L57 (-2.9939, 18.085) -> (-4.1872, 18.1887)
  spline S168 degree 3 poles (-4.1872, 18.1887) (-9.0472, 18.6211) (-11.1573, 19.1227) (-11.2957, 19.901) knots 0 0 0 0 1 1 1 1
  spline S169 degree 3 poles (-11.2957, 19.901) (-11.5032, 20.9733) (-9.3067, 21.5613) (-3.7894, 21.9246) knots 0 0 0 0 1 1 1 1
  spline S170 degree 3 poles (-3.7894, 21.9246) (-1.0568, 22.0975) (6.6743, 21.9937) (8.9054, 21.7343) knots 0 0 0 0 1 1 1 1
  spline S171 degree 3 poles (-2.769, 20.956) (-6.6432, 20.7139) (-9.9293, 20.2642) (-9.6526, 20.0221) knots 0 0 0 0 1 1 1 1
  spline S172 degree 3 poles (-9.6526, 20.0221) (-9.4623, 19.8491) (-7.5771, 19.5378) (-5.8822, 19.4167) knots 0 0 0 0 1 1 1 1
  spline S173 degree 3 poles (-5.8822, 19.4167) (-5.1212, 19.3475) (-4.3256, 19.2784) (-4.1181, 19.2265) knots 0 0 0 0 1 1 1 1
  spline S174 degree 3 poles (-4.1181, 19.2265) (-3.8586, 19.1746) (-3.703, 19.2611) (-3.6338, 19.5205) knots 0 0 0 0 1 1 1 1
  spline S175 degree 3 poles (-3.6338, 19.5205) (-3.5473, 19.7626) (-3.3916, 19.8491) (-3.1495, 19.8145) knots 0 0 0 0 1 1 1 1
  spline S176 degree 3 poles (-3.1495, 19.8145) (-2.6133, 19.7453) (-1.2124, 16.8743) (-0.7281, 14.8507) knots 0 0 0 0 1 1 1 1
  spline S177 degree 3 poles (-0.7281, 14.8507) (-0.3822, 13.4325) (-0.3131, 13.2768) (0.0501, 13.2768) knots 0 0 0 0 1 1 1 1
  spline S178 degree 3 poles (0.0501, 13.2768) (0.4306, 13.2768) (0.4479, 13.3287) (0.3615, 14.1935) knots 0 0 0 0 1 1 1 1
  spline S179 degree 3 poles (0.3615, 14.1935) (0.0329, 17.2894) (-0.1055, 19.3648) (-0.019, 19.5897) knots 0 0 0 0 1 1 1 1
  spline S180 degree 3 poles (-0.019, 19.5897) (0.102, 19.9356) (0.5517, 19.9183) (0.742, 19.5551) knots 0 0 0 0 1 1 1 1
  spline S181 degree 3 poles (0.742, 19.5551) (0.8284, 19.3821) (1.0014, 18.3098) (1.1052, 17.1683) knots 0 0 0 0 1 1 1 1
  spline S182 degree 3 poles (1.1052, 17.1683) (1.4684, 13.1904) (1.4684, 13.2768) (1.8316, 13.2768) knots 0 0 0 0 1 1 1 1
  spline S183 degree 3 poles (1.8316, 13.2768) (2.0045, 13.2768) (2.1602, 13.3287) (2.1602, 13.4152) knots 0 0 0 0 1 1 1 1
  spline S184 degree 3 poles (2.1602, 13.4152) (2.1602, 14.1416) (2.558, 17.5661) (2.679, 17.8774) knots 0 0 0 0 1 1 1 1
  spline S185 degree 3 poles (2.679, 17.8774) (2.852, 18.3271) (3.44, 18.4482) (3.5957, 18.0677) knots 0 0 0 0 1 1 1 1
  spline S186 degree 3 poles (3.5957, 18.0677) (3.6476, 17.9293) (3.613, 17.4969) (3.5438, 17.0645) knots 0 0 0 0 1 1 1 1
  spline S187 degree 3 poles (3.5438, 17.0645) (3.4746, 16.6494) (3.3536, 15.629) (3.2844, 14.7988) knots 0 0 0 0 1 1 1 1
  line L58 (3.2844, 14.7988) -> (3.1633, 13.2768)
  line L59 (3.1633, 13.2768) -> (3.6995, 13.2768)
  spline S188 degree 3 poles (3.6995, 13.2768) (4.1492, 13.2768) (4.2356, 13.346) (4.2356, 13.6746) knots 0 0 0 0 1 1 1 1
  spline S189 degree 3 poles (4.2356, 13.6746) (4.2356, 14.3492) (4.8929, 16.684) (5.3771, 17.7736) knots 0 0 0 0 1 1 1 1
  spline S190 degree 3 poles (5.3771, 17.7736) (5.6193, 18.3271) (6.0517, 18.9843) (6.3284, 19.2611) knots 0 0 0 0 1 1 1 1
  spline S191 degree 3 poles (6.3284, 19.2611) (6.7435, 19.6588) (6.8645, 19.6934) (7.0894, 19.5032) knots 0 0 0 0 1 1 1 1
  spline S192 degree 3 poles (7.0894, 19.5032) (7.2796, 19.3475) (7.7293, 19.3129) (8.7324, 19.3821) knots 0 0 0 0 1 1 1 1
  spline S193 degree 3 poles (8.7324, 19.3821) (10.5139, 19.5205) (12.3645, 19.8491) (12.3645, 20.0221) knots 0 0 0 0 1 1 1 1
  spline S194 degree 3 poles (12.3645, 20.0221) (12.3645, 20.195) (10.6868, 20.5063) (8.5595, 20.7139) knots 0 0 0 0 1 1 1 1
  spline S195 degree 3 poles (8.5595, 20.7139) (6.8127, 20.9041) (-1.0395, 21.0598) (-2.769, 20.956) knots 0 0 0 0 1 1 1 1
  spline S196 degree 3 poles (-3.7203, 12.0662) (-5.9341, 11.8759) (-7.0064, 11.703) (-7.0064, 11.53) knots 0 0 0 0 1 1 1 1
  spline S197 degree 3 poles (-7.0064, 11.53) (-7.0064, 11.4435) (-6.9372, 11.3743) (-6.8507, 11.3743) knots 0 0 0 0 1 1 1 1
  spline S198 degree 3 poles (-6.8507, 11.3743) (-6.7642, 11.3743) (-6.107, 11.3052) (-5.4152, 11.2187) knots 0 0 0 0 1 1 1 1
  spline S199 degree 3 poles (-5.4152, 11.2187) (-4.7234, 11.1322) (-3.4608, 11.0111) (-2.6306, 10.942) knots 0 0 0 0 1 1 1 1
  line L60 (-2.6306, 10.942) -> (-1.1086, 10.8382)
  line L61 (-1.1086, 10.8382) -> (-1.1605, 11.4954)
  spline S200 degree 3 poles (-1.1605, 11.4954) (-1.2297, 12.2564) (-1.2816, 12.2737) (-3.7203, 12.0662) knots 0 0 0 0 1 1 1 1
  spline S201 degree 3 poles (-0.0363, 10.6479) (0.0329, 9.7659) (0.0674, 8.7454) (0.0329, 8.3995) knots 0 0 0 0 1 1 1 1
  spline S202 degree 3 poles (0.0329, 8.3995) (-0.0536, 7.7769) (-0.0363, 7.7596) (0.6036, 7.6558) knots 0 0 0 0 1 1 1 1
  spline S203 degree 3 poles (0.6036, 7.6558) (1.4857, 7.5002) (1.9872, 7.8288) (1.9872, 8.5379) knots 0 0 0 0 1 1 1 1
  spline S204 degree 3 poles (1.9872, 8.5379) (1.9872, 8.8319) (2.0391, 9.7832) (2.091, 10.6479) knots 0 0 0 0 1 1 1 1
  spline S205 degree 3 poles (2.091, 10.6479) (2.2121, 12.1872) (2.1948, 12.2391) (1.8316, 12.2391) knots 0 0 0 0 1 1 1 1
  spline S206 degree 3 poles (1.8316, 12.2391) (1.5203, 12.2391) (1.4684, 12.1353) (1.4684, 11.5646) knots 0 0 0 0 1 1 1 1
  spline S207 degree 3 poles (1.4684, 11.5646) (1.4684, 10.769) (1.0879, 10.3539) (0.6901, 10.6825) knots 0 0 0 0 1 1 1 1
  spline S208 degree 3 poles (0.6901, 10.6825) (0.5344, 10.8036) (0.4306, 11.1841) (0.4306, 11.5646) knots 0 0 0 0 1 1 1 1
  spline S209 degree 3 poles (0.4306, 11.5646) (0.4306, 12.1008) (0.3615, 12.2391) (0.1193, 12.2391) knots 0 0 0 0 1 1 1 1
  spline S210 degree 3 poles (0.1193, 12.2391) (-0.1574, 12.2391) (-0.1747, 12.1181) (-0.0363, 10.6479) knots 0 0 0 0 1 1 1 1
  spline S211 degree 3 poles (3.1287, 11.703) (3.0768, 11.4089) (3.025, 10.5096) (3.025, 9.714) knots 0 0 0 0 1 1 1 1
  spline S212 degree 3 poles (3.025, 9.714) (3.025, 8.3822) (3.0595, 8.2612) (3.3709, 8.2612) knots 0 0 0 0 1 1 1 1
  spline S213 degree 3 poles (3.3709, 8.2612) (3.6649, 8.2612) (3.7168, 8.3822) (3.7168, 9.0914) knots 0 0 0 0 1 1 1 1
  spline S214 degree 3 poles (3.7168, 9.0914) (3.7168, 9.541) (3.7687, 10.4231) (3.8378, 11.0803) knots 0 0 0 0 1 1 1 1
  spline S215 degree 3 poles (3.8378, 11.0803) (3.9243, 12.1699) (3.9243, 12.2391) (3.5957, 12.2391) knots 0 0 0 0 1 1 1 1
  spline S216 degree 3 poles (3.5957, 12.2391) (3.3363, 12.2391) (3.2152, 12.0835) (3.1287, 11.703) knots 0 0 0 0 1 1 1 1
  spline S217 degree 3 poles (4.9966, 12.0835) (4.962, 12.0489) (4.9275, 11.7548) (4.9275, 11.4435) knots 0 0 0 0 1 1 1 1
  spline S218 degree 3 poles (4.9275, 11.4435) (4.9275, 10.9074) (4.962, 10.8728) (5.4117, 10.942) knots 0 0 0 0 1 1 1 1
  spline S219 degree 3 poles (5.4117, 10.942) (5.6712, 10.9766) (6.5359, 11.063) (7.3488, 11.1149) knots 0 0 0 0 1 1 1 1
  spline S220 degree 3 poles (7.3488, 11.1149) (9.2167, 11.236) (10.1161, 11.3916) (10.1161, 11.5473) knots 0 0 0 0 1 1 1 1
  spline S221 degree 3 poles (10.1161, 11.5473) (10.1161, 11.7548) (5.1869, 12.2737) (4.9966, 12.0835) knots 0 0 0 0 1 1 1 1
  spline S222 degree 3 poles (-3.5473, 7.258) (-4.3429, 6.8775) (-4.3083, 6.5835) (-3.4435, 6.203) knots 0 0 0 0 1 1 1 1
  line L62 (-3.4435, 6.203) -> (-2.7344, 5.8744)
  line L63 (-2.7344, 5.8744) -> (-2.2674, 6.4797)
  spline S223 degree 3 poles (-2.2674, 6.4797) (-1.9907, 6.8084) (-1.8178, 7.1024) (-1.8524, 7.1197) knots 0 0 0 0 1 1 1 1
  spline S224 degree 3 poles (-1.8524, 7.1197) (-1.9907, 7.258) (-2.6825, 7.5694) (-2.8036, 7.5694) knots 0 0 0 0 1 1 1 1
  spline S225 degree 3 poles (-2.8036, 7.5694) (-2.8728, 7.5694) (-3.2187, 7.431) (-3.5473, 7.258) knots 0 0 0 0 1 1 1 1
  spline S226 degree 3 poles (2.5061, 7.1024) (2.5061, 7.0505) (2.6272, 6.8602) (2.7828, 6.6873) knots 0 0 0 0 1 1 1 1
  spline S227 degree 3 poles (2.7828, 6.6873) (3.0077, 6.4452) (3.1287, 6.4106) (3.4746, 6.5662) knots 0 0 0 0 1 1 1 1
  spline S228 degree 3 poles (3.4746, 6.5662) (3.786, 6.7219) (3.8378, 6.8084) (3.6995, 6.9986) knots 0 0 0 0 1 1 1 1
  spline S229 degree 3 poles (3.6995, 6.9986) (3.4919, 7.2234) (2.5061, 7.3272) (2.5061, 7.1024) knots 0 0 0 0 1 1 1 1
  spline S230 degree 3 poles (-0.3304, 6.5316) (-0.9876, 6.3241) (-1.6275, 5.7187) (-1.9215, 5.0269) knots 0 0 0 0 1 1 1 1
  spline S231 degree 3 poles (-1.9215, 5.0269) (-2.2674, 4.2313) (-2.2329, 4.1449) (-1.5929, 3.8681) knots 0 0 0 0 1 1 1 1
  spline S232 degree 3 poles (-1.5929, 3.8681) (-0.8146, 3.5568) (-0.192, 2.7612) (-0.4514, 2.4499) knots 0 0 0 0 1 1 1 1
  spline S233 degree 3 poles (-0.4514, 2.4499) (-0.7281, 2.104) (-0.9184, 2.1386) (-1.5064, 2.6402) knots 0 0 0 0 1 1 1 1
  spline S234 degree 3 poles (-1.5064, 2.6402) (-2.2328, 3.2455) (-3.0803, 3.2282) (-3.7376, 2.571) knots 0 0 0 0 1 1 1 1
  spline S235 degree 3 poles (-3.7376, 2.571) (-4.0143, 2.2943) (-4.2391, 1.9483) (-4.2391, 1.81) knots 0 0 0 0 1 1 1 1
  spline S236 degree 3 poles (-4.2391, 1.81) (-4.2391, 1.4295) (-4.7753, 1.2911) (-5.0693, 1.5851) knots 0 0 0 0 1 1 1 1
  spline S237 degree 3 poles (-5.0693, 1.5851) (-5.4671, 1.9829) (-4.7753, 3.2455) (-3.8932, 3.7471) knots 0 0 0 0 1 1 1 1
  spline S238 degree 3 poles (-3.8932, 3.7471) (-2.6479, 4.4389) (-3.2187, 5.4939) (-4.8445, 5.4939) knots 0 0 0 0 1 1 1 1
  spline S239 degree 3 poles (-4.8445, 5.4939) (-5.8476, 5.4939) (-7.1966, 4.6291) (-6.574, 4.387) knots 0 0 0 0 1 1 1 1
  spline S240 degree 3 poles (-6.574, 4.387) (-6.401, 4.3351) (-6.3146, 4.1276) (-6.3492, 3.9027) knots 0 0 0 0 1 1 1 1
  spline S241 degree 3 poles (-6.3492, 3.9027) (-6.401, 3.5568) (-6.4875, 3.5049) (-7.0929, 3.5568) knots 0 0 0 0 1 1 1 1
  spline S242 degree 3 poles (-7.0929, 3.5568) (-8.7186, 3.6606) (-9.7045, 3.1071) (-10.2233, 1.7581) knots 0 0 0 0 1 1 1 1
  spline S243 degree 3 poles (-10.2233, 1.7581) (-10.4655, 1.1009) (-10.4828, 0.876) (-10.3098, 0.3053) knots 0 0 0 0 1 1 1 1
  spline S244 degree 3 poles (-10.3098, 0.3053) (-10.0158, -0.6633) (-9.0645, -1.5626) (-8.2171, -1.701) knots 0 0 0 0 1 1 1 1
  spline S245 degree 3 poles (-8.2171, -1.701) (-7.3869, -1.8394) (-7.041, -2.168) (-7.3523, -2.5312) knots 0 0 0 0 1 1 1 1
  spline S246 degree 3 poles (-7.3523, -2.5312) (-7.4561, -2.6695) (-7.7155, -2.8079) (-7.923, -2.8425) knots 0 0 0 0 1 1 1 1
  spline S247 degree 3 poles (-7.923, -2.8425) (-8.3035, -2.8944) (-8.3035, -2.8944) (-7.8366, -3.3613) knots 0 0 0 0 1 1 1 1
  spline S248 degree 3 poles (-7.8366, -3.3613) (-7.4734, -3.7246) (-7.1966, -3.8456) (-6.6778, -3.8456) knots 0 0 0 0 1 1 1 1
  line L64 (-6.6778, -3.8456) -> (-5.9687, -3.8456)
  line L65 (-5.9687, -3.8456) -> (-6.3319, -3.1711)
  spline S249 degree 3 poles (-6.3319, -3.1711) (-6.7988, -2.2544) (-6.7297, -1.5107) (-6.1416, -1.5107) knots 0 0 0 0 1 1 1 1
  spline S250 degree 3 poles (-6.1416, -1.5107) (-5.7957, -1.5107) (-5.7092, -1.6145) (-5.6055, -2.1161) knots 0 0 0 0 1 1 1 1
  spline S251 degree 3 poles (-5.6055, -2.1161) (-5.5363, -2.4447) (-5.2595, -2.8944) (-5.0001, -3.1192) knots 0 0 0 0 1 1 1 1
  spline S252 degree 3 poles (-5.0001, -3.1192) (-4.6196, -3.4651) (-4.3775, -3.517) (-3.5646, -3.4651) knots 0 0 0 0 1 1 1 1
  spline S253 degree 3 poles (-3.5646, -3.4651) (-2.6825, -3.4132) (-2.5961, -3.4478) (-2.5442, -3.7764) knots 0 0 0 0 1 1 1 1
  spline S254 degree 3 poles (-2.5442, -3.7764) (-2.475, -4.278) (-3.3052, -4.6066) (-4.3083, -4.5028) knots 0 0 0 0 1 1 1 1
  spline S255 degree 3 poles (-4.3083, -4.5028) (-5.7611, -4.3299) (-5.813, -4.9525) (-4.4121, -5.6962) knots 0 0 0 0 1 1 1 1
  spline S256 degree 3 poles (-4.4121, -5.6962) (-3.5646, -6.1459) (-2.4404, -6.2151) (-1.5929, -5.8519) knots 0 0 0 0 1 1 1 1
  spline S257 degree 3 poles (-1.5929, -5.8519) (-0.9876, -5.6098) (0.0847, -4.5028) (0.0847, -4.1223) knots 0 0 0 0 1 1 1 1
  spline S258 degree 3 poles (0.0847, -4.1223) (0.0847, -3.7764) (0.5171, -3.4824) (0.8457, -3.6035) knots 0 0 0 0 1 1 1 1
  spline S259 degree 3 poles (0.8457, -3.6035) (1.1916, -3.7418) (1.1916, -4.2261) (0.8457, -4.9179) knots 0 0 0 0 1 1 1 1
  spline S260 degree 3 poles (0.8457, -4.9179) (0.5863, -5.4195) (0.5863, -5.4714) (0.863, -5.6789) knots 0 0 0 0 1 1 1 1
  spline S261 degree 3 poles (0.863, -5.6789) (1.2608, -5.973) (2.7136, -6.1459) (3.4055, -6.0075) knots 0 0 0 0 1 1 1 1
  spline S262 degree 3 poles (3.4055, -6.0075) (3.7168, -5.9384) (4.2702, -5.7308) (4.6334, -5.5406) knots 0 0 0 0 1 1 1 1
  spline S263 degree 3 poles (4.6334, -5.5406) (5.2907, -5.212) (5.2907, -5.1947) (4.9966, -4.866) knots 0 0 0 0 1 1 1 1
  spline S264 degree 3 poles (4.9966, -4.866) (4.841, -4.6931) (4.5124, -4.5374) (4.2875, -4.5374) knots 0 0 0 0 1 1 1 1
  spline S265 degree 3 poles (4.2875, -4.5374) (3.7687, -4.5374) (2.8347, -4.1396) (2.5407, -3.811) knots 0 0 0 0 1 1 1 1
  spline S266 degree 3 poles (2.5407, -3.811) (2.2813, -3.4824) (2.4369, -2.9808) (2.8347, -2.9808) knots 0 0 0 0 1 1 1 1
  spline S267 degree 3 poles (2.8347, -2.9808) (2.9904, -2.9808) (3.2671, -3.1019) (3.44, -3.2403) knots 0 0 0 0 1 1 1 1
  spline S268 degree 3 poles (3.44, -3.2403) (4.2875, -3.8802) (5.9479, -3.2576) (6.2073, -2.2026) knots 0 0 0 0 1 1 1 1
  spline S269 degree 3 poles (6.2073, -2.2026) (6.2765, -1.9258) (6.4322, -1.7702) (6.6743, -1.7702) knots 0 0 0 0 1 1 1 1
  spline S270 degree 3 poles (6.6743, -1.7702) (7.4526, -1.7702) (7.2796, -2.929) (6.3803, -3.7937) knots 0 0 0 0 1 1 1 1
  line L66 (6.3803, -3.7937) -> (5.7749, -4.3472)
  line L67 (5.7749, -4.3472) -> (6.3284, -4.6412)
  spline S271 degree 3 poles (6.3284, -4.6412) (7.1931, -5.0736) (8.5941, -4.9006) (9.2686, -4.2607) knots 0 0 0 0 1 1 1 1
  spline S272 degree 3 poles (9.2686, -4.2607) (9.7702, -3.7937) (9.7702, -3.7591) (9.4243, -3.6381) knots 0 0 0 0 1 1 1 1
  spline S273 degree 3 poles (9.4243, -3.6381) (9.1648, -3.5516) (9.0783, -3.3786) (9.1129, -3.1192) knots 0 0 0 0 1 1 1 1
  spline S274 degree 3 poles (9.1129, -3.1192) (9.1648, -2.756) (9.2513, -2.7214) (9.9604, -2.7733) knots 0 0 0 0 1 1 1 1
  spline S275 degree 3 poles (9.9604, -2.7733) (11.3959, -2.8598) (12.2953, -1.7183) (11.7764, -0.473) knots 0 0 0 0 1 1 1 1
  spline S276 degree 3 poles (11.7764, -0.473) (11.6381, -0.1444) (11.3959, 0.1842) (11.2403, 0.2361) knots 0 0 0 0 1 1 1 1
  spline S277 degree 3 poles (11.2403, 0.2361) (11.1019, 0.288) (10.9808, 0.5301) (10.9808, 0.755) knots 0 0 0 0 1 1 1 1
  spline S278 degree 3 poles (10.9808, 0.755) (10.9808, 1.3603) (11.6554, 1.3084) (12.278, 0.6512) knots 0 0 0 0 1 1 1 1
  spline S279 degree 3 poles (12.278, 0.6512) (12.8487, 0.0459) (13.0563, 0.1842) (13.0563, 1.2219) knots 0 0 0 0 1 1 1 1
  spline S280 degree 3 poles (13.0563, 1.2219) (13.0563, 1.9829) (12.8487, 2.4326) (12.2261, 3.1071) knots 0 0 0 0 1 1 1 1
  spline S281 degree 3 poles (12.2261, 3.1071) (11.3959, 4.0065) (9.8566, 3.8854) (9.0092, 2.8823) knots 0 0 0 0 1 1 1 1
  spline S282 degree 3 poles (9.0092, 2.8823) (8.2655, 2.0002) (7.5218, 2.4326) (8.1098, 3.4185) knots 0 0 0 0 1 1 1 1
  spline S283 degree 3 poles (8.1098, 3.4185) (8.2655, 3.6952) (8.3865, 3.9892) (8.3865, 4.093) knots 0 0 0 0 1 1 1 1
  spline S284 degree 3 poles (8.3865, 4.093) (8.3865, 4.4216) (7.2796, 5.5458) (6.7089, 5.7706) knots 0 0 0 0 1 1 1 1
  spline S285 degree 3 poles (6.7089, 5.7706) (6.0516, 6.0474) (4.8583, 6.082) (4.4086, 5.8398) knots 0 0 0 0 1 1 1 1
  spline S286 degree 3 poles (4.4086, 5.8398) (4.0973, 5.6669) (4.0973, 5.6323) (4.5124, 5.0269) knots 0 0 0 0 1 1 1 1
  spline S287 degree 3 poles (4.5124, 5.0269) (5.0485, 4.2313) (5.0312, 3.332) (4.4951, 3.332) knots 0 0 0 0 1 1 1 1
  spline S288 degree 3 poles (4.4951, 3.332) (4.2529, 3.332) (4.0973, 3.5049) (3.9589, 3.92) knots 0 0 0 0 1 1 1 1
  spline S289 degree 3 poles (3.9589, 3.92) (3.5784, 5.1307) (2.2985, 5.5285) (1.2781, 4.7675) knots 0 0 0 0 1 1 1 1
  spline S290 degree 3 poles (1.2781, 4.7675) (0.8111, 4.4216) (0.742, 4.4043) (0.4998, 4.6637) knots 0 0 0 0 1 1 1 1
  spline S291 degree 3 poles (0.4998, 4.6637) (0.1193, 5.0442) (0.4133, 5.5285) (1.2262, 5.9263) knots 0 0 0 0 1 1 1 1
  spline S292 degree 3 poles (1.2262, 5.9263) (1.6932, 6.1511) (1.797, 6.2722) (1.624, 6.3587) knots 0 0 0 0 1 1 1 1
  spline S293 degree 3 poles (1.624, 6.3587) (1.1916, 6.6008) (0.1885, 6.6873) (-0.3304, 6.5316) knots 0 0 0 0 1 1 1 1
  spline S294 degree 3 poles (8.6979, 6.2203) (8.3001, 6.1338) (8.3001, 6.0992) (8.8535, 5.3555) knots 0 0 0 0 1 1 1 1
  spline S295 degree 3 poles (8.8535, 5.3555) (9.1129, 5.0096) (9.3378, 4.6983) (9.3551, 4.6637) knots 0 0 0 0 1 1 1 1
  spline S296 degree 3 poles (9.3551, 4.6637) (9.4589, 4.5081) (10.6349, 4.8713) (10.6349, 5.0615) knots 0 0 0 0 1 1 1 1
  spline S297 degree 3 poles (10.6349, 5.0615) (10.6349, 5.6842) (9.4588, 6.3933) (8.6979, 6.2203) knots 0 0 0 0 1 1 1 1
  spline S298 degree 3 poles (-8.1133, 5.6669) (-8.4073, 5.4939) (-8.7359, 5.1307) (-8.8743, 4.8713) knots 0 0 0 0 1 1 1 1
  line L68 (-8.8743, 4.8713) -> (-9.1164, 4.4043)
  line L69 (-9.1164, 4.4043) -> (-8.5457, 4.5254)
  spline S299 degree 3 poles (-8.5457, 4.5254) (-8.2171, 4.5772) (-7.923, 4.7329) (-7.8885, 4.854) knots 0 0 0 0 1 1 1 1
  spline S300 degree 3 poles (-7.8885, 4.854) (-7.8539, 4.9577) (-7.5944, 5.2691) (-7.335, 5.5285) knots 0 0 0 0 1 1 1 1
  spline S301 degree 3 poles (-7.335, 5.5285) (-6.8853, 5.9955) (-6.868, 6.0128) (-7.2312, 6.0128) knots 0 0 0 0 1 1 1 1
  spline S302 degree 3 poles (-7.2312, 6.0128) (-7.4388, 6.0128) (-7.8366, 5.8571) (-8.1133, 5.6669) knots 0 0 0 0 1 1 1 1
  spline S303 degree 3 poles (10.8771, -3.7937) (10.6522, -4.0359) (10.4966, -4.278) (10.5485, -4.3299) knots 0 0 0 0 1 1 1 1
  spline S304 degree 3 poles (10.5485, -4.3299) (10.6868, -4.4683) (11.4997, -3.8456) (11.4997, -3.5862) knots 0 0 0 0 1 1 1 1
  spline S305 degree 3 poles (11.4997, -3.5862) (11.4997, -3.223) (11.3613, -3.2576) (10.8771, -3.7937) knots 0 0 0 0 1 1 1 1
  spline S306 degree 3 poles (-7.0237, -5.2293) (-6.5048, -5.6789) (-6.2454, -5.6789) (-6.4875, -5.2293) knots 0 0 0 0 1 1 1 1
  spline S307 degree 3 poles (-6.4875, -5.2293) (-6.5913, -5.039) (-6.8507, -4.8833) (-7.0583, -4.8833) knots 0 0 0 0 1 1 1 1
  line L70 (-7.0583, -4.8833) -> (-7.4388, -4.9006)
  line L71 (-7.4388, -4.9006) -> (-7.0237, -5.2293)
  line L72 (-1.0222, -6.6129) -> (-1.5064, -6.9242)
  line L73 (-1.5064, -6.9242) -> (-1.0741, -7.2009)
  spline S308 degree 3 poles (-1.0741, -7.2009) (-0.4168, -7.6506) (0.4479, -7.7198) (1.2089, -7.4085) knots 0 0 0 0 1 1 1 1
  spline S309 degree 3 poles (1.2089, -7.4085) (1.5721, -7.2528) (1.8143, -7.0799) (1.7624, -7.0107) knots 0 0 0 0 1 1 1 1
  spline S310 degree 3 poles (1.7624, -7.0107) (1.624, -6.8723) (-0.1228, -6.2843) (-0.3477, -6.2843) knots 0 0 0 0 1 1 1 1
  spline S311 degree 3 poles (-0.3477, -6.2843) (-0.4341, -6.2843) (-0.7454, -6.4399) (-1.0222, -6.6129) knots 0 0 0 0 1 1 1 1
extrude "Extrude1" add sketch "Sketch2" along normal blind 3 contours S121 S122 S123 S124 S125 S126 S127 S128 S129 L50 L51 S130 S131 S132 S133 S134 S135 S136 S137 S138 S139 S140 S141 S142 S143 S144 S145 S146 S147 S148 S149 S150 S151 S152 S153 S154 S155 S156 S157 S158 S159 S160 S161 S162 L52 L53 L54 L55 S163 S164 S165 S166 S167 L56 L57 S168 S169 S170 makes body 1
extrude "Extrude2" add sketch "Sketch1" along normal blind 5 separate body makes body 2